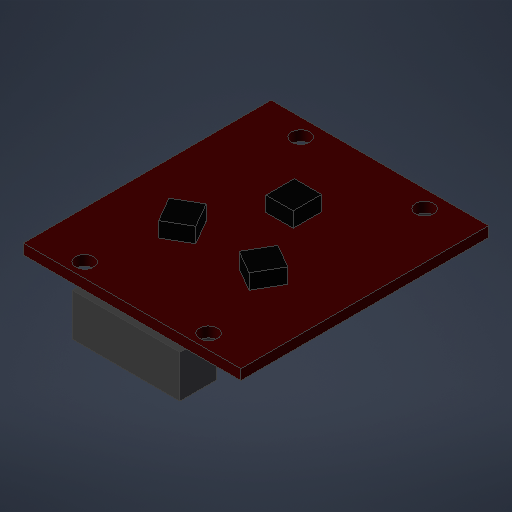
# Autodesk Inventor part: Spectral_Sensor
Saved by Autodesk Inventor 2026 (Build 300175000, 175)
## iProperties
Created: 2025-04-13
Part Number: Spectral_Sensor
Material: Generic
Document SubType Name: Modeling
Designer: ct_vi
Density: 1 g/cm^3
Appearance: Default
Author: ct_vi
Autodesk Inventor part; units mm, degrees
ref_plane "YZ Plane" through (0, 0, 0) normal (1, 0, 0) x (0, 1, 0)
ref_plane "XZ Plane" through (0, 0, 0) normal (0, 1, 0) x (-1, 0, 0)
ref_plane "XY Plane" through (0, 0, 0) normal (0, 0, 1) x (1, 0, 0)
sketch "Sketch1" plane through (0, 0, 0) normal (0, 1, 0) x (-1, 0, 0)
  line L0 (-18.0542, -22.0034) -> (17.9458, -22.0034)
  line L1 (17.9458, -22.0034) -> (17.9458, 18.9966)
  line L2 (17.9458, 18.9966) -> (-18.0542, 18.9966)
  line L3 (-18.0542, 18.9966) -> (-18.0542, -22.0034)
  line L4 (-18.0542, 18.9966) -> (-0.0043, 18.9966)
  line L5 (-18.0043, 0.0465) -> (-18.0542, 18.9966)
  circle A0 centre (0, 0) radius 11.5
  circle A1 centre (0, 0) radius 12.5
  line L6 (-2.2543, -5.4535) -> (-2.2543, -10.1535)
  line L7 (-2.2543, -10.1535) -> (2.2457, -10.1535)
  line L8 (2.2457, -10.1535) -> (2.2457, -5.4535)
  line L9 (2.2457, -5.4535) -> (-2.2543, -5.4535)
  line L10 (5.9338, 0.7614) -> (9.8309, 3.0114)
  line L11 (9.8309, 3.0114) -> (7.4809, 7.0817)
  line L12 (7.4809, 7.0817) -> (3.5838, 4.8317)
  line L13 (5.9338, 0.7614) -> (3.5838, 4.8317)
  line L14 (-3.5925, 4.8317) -> (-7.4896, 7.0817)
  line L15 (-7.4896, 7.0817) -> (-9.8396, 3.0114)
  line L16 (-9.8396, 3.0114) -> (-5.9425, 0.7614)
  line L17 (-3.5925, 4.8317) -> (-5.9425, 0.7614)
  circle A2 centre (10.1947, -19.139) radius 1.5
  circle A3 centre (-10.3053, 16.611) radius 1.5
  circle A4 centre (10.1947, 16.611) radius 1.5
  circle A5 centre (-10.3053, -19.139) radius 1.5
  line L18 (18.9458, -23.0034) -> (-19.0542, -23.0034)
  line L19 (-19.0542, -23.0034) -> (-19.0542, 19.9966)
  line L20 (-19.0542, 19.9966) -> (18.9458, 19.9966)
  line L21 (18.9458, 19.9966) -> (18.9458, -23.0034)
  line L22 (18.9458, -23.0034) -> (-18.9686, -22.7989) construction
  line L23 (-18.9686, -22.7989) -> (-18.7366, 20.211) construction
  line L24 (-18.7366, 20.211) -> (19.1777, 20.0065) construction
  line L25 (19.1777, 20.0065) -> (18.9458, -23.0034) construction
  point P0 (-0.0043, -1.4535)
  dimension "d0" = 41
  dimension "d1" = 36
  dimension "d2" = 4.7
  dimension "d3" = 4.5
  dimension "d4" = 4.5
  dimension "d5" = 4.7
  dimension "d6" = 3
  dimension "d7" = 3
  dimension "d8" = 3
  dimension "d9" = 3
  dimension "d10" = 1
  constraints: 44 end point, 8 perpendicular, 6 centre point, 4 parallel, 3 horizontal, 2 coincident, 1 point on line, 5 other
  measures "d0" distance of L1.start L2.start
  measures "d1" distance of L3.end L1.start
  measures "d2" distance of L9.end L7.start
  measures "d3" distance of L7.start L8.start
  measures "d4" distance of L13.start L10.end
  measures "d5" distance of L10.end L12.start
  measures "d6" diameter of A2
  measures "d7" diameter of A3
  measures "d8" diameter of A4
  measures "d9" diameter of A5
  measures "d10" distance between parallel lines of L0 L18
extrude "Extrusion1" add sketch "Sketch1" against normal blind 1.7 contours L3 L2 L1 L0 | A0 | A1 | L9 L8 L7 L6 | L13 L12 L11 L10 | L17 L16 L15 L14
extrude "Extrusion2" add sketch "Sketch1" along normal blind 2.5 contours L9 L8 L7 L6 | L13 L12 L11 L10 | L17 L16 L15 L14
sketch "Sketch2" plane through (0, -1.7, 0) normal (0, -1, 0) x (1, 0, 0)
  line L0 (18.0542, 18.9966) -> (-17.9458, 18.9966) projected
  line L1 (8.9542, 19.9966) -> (-8.8458, 19.9966)
  line L2 (-8.8458, 19.9966) -> (-8.8458, 13.9966)
  line L3 (-8.8458, 13.9966) -> (8.9542, 13.9966)
  line L4 (8.9542, 13.9966) -> (8.9542, 19.9966)
  line L5 (18.0542, -22.0034) -> (-17.9458, -22.0034) projected
  line L6 (0.0542, -22.0034) -> (0.0542, -23.0034)
  line L7 (-8.8458, -23.0034) -> (8.9542, -23.0034)
  line L8 (8.9542, -23.0034) -> (8.9542, -17.0034)
  line L9 (8.9542, -17.0034) -> (-8.8458, -17.0034)
  line L10 (-8.8458, -17.0034) -> (-8.8458, -23.0034)
  point P0 (0, 0)
  dimension "d50" = 17.8
  dimension "d51" = 6
  dimension "d54" = 1
  dimension "d56" = 17.8
  dimension "d57" = 6
  constraints: 18 end point, 4 parallel, 2 horizontal, 2 perpendicular, 1 midpoint, 1 vertical
  measures "d50" distance of L3.end L2.end
  measures "d51" distance of L2.end L1.end
  measures "d54" distance of L6.start L6.end
  measures "d56" distance of L9.end L8.end
  measures "d57" distance of L8.end L7.end
extrude "Extrusion3" add sketch "Sketch2" along normal blind 7
body "Solid1"
